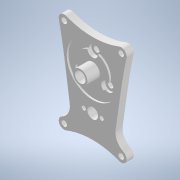
# Autodesk Inventor part: Adapterlowerplate
Saved by Autodesk Inventor 2022 (Build 260153070, 153G)
## iProperties
Created: 2021-10-27
Part Number: Adapterlowerplate
Material: Generic
Document SubType Name: Modeling
Designer: a laptop
Density: 1 g/cm^3
Appearance: Default
Author: a laptop
Autodesk Inventor part; units mm, degrees
ref_plane "YZ Plane" through (0, 0, 0) normal (1, 0, 0) x (0, 1, 0)
ref_plane "XZ Plane" through (0, 0, 0) normal (0, 1, 0) x (-1, 0, 0)
ref_plane "XY Plane" through (0, 0, 0) normal (0, 0, 1) x (1, 0, 0)
sketch "Sketch1" plane through (0, 0, 0) normal (0, 0, 1) x (1, 0, 0)
  circle A0 centre (4.7942, 16.5) radius 1.6 projected
  circle A1 centre (-3, 30) radius 1.6 projected
  circle A2 centre (-10.7942, 16.5) radius 1.6 projected
  circle A3 centre (2, 0) radius 1.15 projected
  circle A4 centre (-3, 0) radius 3 projected
  circle A5 centre (-8, 0) radius 1.15 projected
  circle A6 centre (-3, 0) radius 9 construction
  circle A7 centre (-3, 21) radius 12 construction
  circle A8 centre (-3, 21) radius 6
  circle A9 centre (-3, 21) radius 16 construction
  circle A10 centre (-3, 0) radius 13 construction
  line L0 (12.8359, 18.7143) -> (9.8667, -1.8571)
  line L1 (-18.8359, 18.7143) -> (-15.8667, -1.8571)
  circle A11 centre (13, 37) radius 3.05
  circle A12 centre (13, 37) radius 1.55
  circle A13 centre (13, -13) radius 3.05
  circle A14 centre (13, -13) radius 1.55
  circle A15 centre (-19, -13) radius 3.05
  circle A16 centre (-19, -13) radius 1.55
  circle A17 centre (-19, 37) radius 3.05
  circle A18 centre (-19, 37) radius 1.55
  arc A19 (-3, 37) -> (11.878, 39.8361) centre (-3, 77.4422) ccw
  arc A20 (-17.878, 39.8361) -> (-3, 37) centre (-3, 77.4422) ccw
  arc A21 (11.878, -15.8361) -> (-3, -13) centre (-3, -53.4422) ccw
  arc A22 (-3, -13) -> (-17.878, -15.8361) centre (-3, -53.4422) ccw
  arc A23 (15.9833, 36.3655) -> (12.8359, 18.7143) centre (280.8872, -19.9756) ccw
  arc A24 (9.8667, -1.8571) -> (14.3284, -10.2545) centre (17.8351, -3.0073) ccw
  arc A25 (-20.3284, -10.2545) -> (-15.8667, -1.8571) centre (-23.8351, -3.0073) ccw
  arc A26 (-18.8359, 18.7143) -> (-21.9833, 36.3655) centre (-286.8872, -19.9756) ccw
  point P0 (0, 0)
  point P1 (-3, -13)
  dimension "d0" = 12
  dimension "d1" = 4
  dimension "d2" = 4
  dimension "d3" = 3.1
  dimension "d4" = 1.5
  dimension "d5" = 3.1
  dimension "d6" = 1.5
  dimension "d7" = 3.1
  dimension "d8" = 1.5
  dimension "d9" = 3.1
  dimension "d10" = 1.5
  dimension "d11" = 32
  dimension "d12" = 50
  dimension "d14" = 50
  dimension "d19" = 16
  dimension "d20" = 37
  constraints: 31 point on circle, 20 tangent, 19 centre point, 8 coincident, 4 end point, 3 horizontal alignment, 3 vertical alignment
  measures "d0" diameter of A8
  measures "d1" radial gap between concentric circles of A7 A9
  measures "d2" radial gap between concentric circles of A6 A10
  measures "d3" diameter of A12
  measures "d4" radial gap between concentric circles of A11 A12
  measures "d5" diameter of A14
  measures "d6" radial gap between concentric circles of A13 A14
  measures "d7" diameter of A16
  measures "d8" radial gap between concentric circles of A15 A16
  measures "d9" diameter of A18
  measures "d10" radial gap between concentric circles of A17 A18
  measures "d11" distance of A18.centre A11.centre
  measures "d12" distance of A14.centre A11.centre
  measures "d14" distance of A17.centre A16.centre
  measures "d19" horizontal distance of A11.centre A1.centre
  measures "d20" vertical distance of point (-3, 0) A11.centre
extrude "Extrusion1" add sketch "Sketch1" along normal blind 4
sketch "Sketch2" plane through (0, 0, 4) normal (0, 0, 1) x (1, 0, 0)
  circle A0 centre (-3, 21) radius 4 projected
  circle A1 centre (-3, 21) radius 6 projected
  circle A2 centre (-3, 21) radius 2.5 construction
  circle A3 centre (-3, 21) radius 3
  point P0 (0, 0)
  dimension "d21" = 1
  constraints: 1 centre point, 1 coincident
  measures "d21" radial gap between concentric circles of A0 A3
extrude "Extrusion2" add sketch "Sketch2" against normal blind 2 contours A0 | A1
extrude "Extrusion3" add sketch "Sketch2" along normal blind 7 contours A0
sketch "Sketch3" plane through (0, 0, 4) normal (0, 0, 1) x (1, 0, 0)
  circle A0 centre (-3, 21) radius 11.05 construction
  circle A1 centre (-3, 21) radius 9.3
  circle A2 centre (-3, 21) radius 14.55
  circle A3 centre (-3, 21) radius 3 projected
  point P0 (0, 0)
  dimension "d26" = 1.75
  dimension "d27" = 3.5
  constraints: 3 centre point
  measures "d26" radial gap between concentric circles of A1 A0
  measures "d27" radial gap between concentric circles of A2 A0
extrude "Extrusion4" cut sketch "Sketch3" against normal blind 1 contours A2
sketch "Sketch4" plane through (0, 0, 4) normal (0, 0, 1) x (1, 0, 0)
  arc A0 (-1.4083, 30.1628) -> (-4.5917, 30.1628) centre (-3, 30) ccw projected
  arc A1 (-4.5917, 30.1628) -> (-1.4083, 30.1628) centre (-3, 30) ccw projected
  circle A2 centre (-3, 30) radius 3
  circle A3 centre (-3, 21) radius 6 projected
  circle A4 centre (-10.7942, 16.5) radius 3
  circle A5 centre (4.7942, 16.5) radius 3
  point P0 (0, 0)
  dimension "d32" = 360
  constraints: 3 centre point, 1 coincident, 1 tangent, 7 other
extrude "Extrusion5" cut sketch "Sketch4" against normal blind 2.25 contours A1 A0 | A2 | A5 | A4
body "Solid1"
